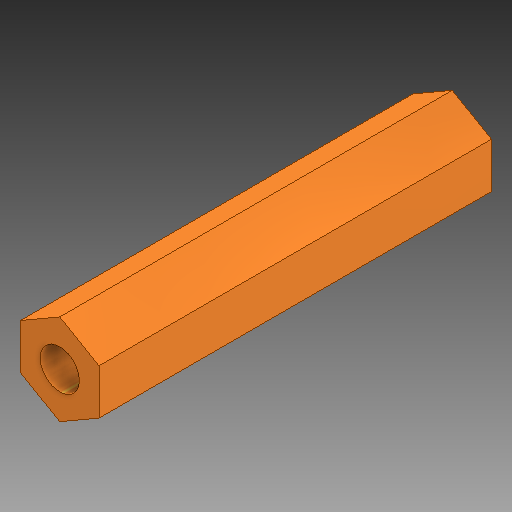
# Autodesk Inventor part: Стойка м3х40
Saved by Autodesk Inventor 2022 (Build 260153000, 153)
## iProperties
Created: 2025-01-23
Part Number: Стойка м3х40
Material: Типовые
Document SubType Name: Modeling
Designer: Ivan
Density: 1 g/cm^3
Appearance: Металл — 1600F
Mass: 0.72325 g
Surface Area: 9.54498 cm^2
Volume: 0.72325 cm^3
Author: Ivan
Title: Стойка м3х40
Autodesk Inventor part; units mm, degrees
ref_plane "YZ Plane" through (0, 0, 0) normal (1, 0, 0) x (0, 1, 0)
ref_plane "XZ Plane" through (0, 0, 0) normal (0, 1, 0) x (-1, 0, 0)
ref_plane "XY Plane" through (0, 0, 0) normal (0, 0, 1) x (1, 0, 0)
sketch "Эскиз1" plane through (0, 0, 0) normal (0, 0, 1) x (1, 0, 0)
  line L0 (0, 3.4641) -> (3, 1.7321)
  line L1 (3, 1.7321) -> (3, -1.7321)
  line L2 (3, -1.7321) -> (0, -3.4641)
  line L3 (0, -3.4641) -> (-3, -1.7321)
  line L4 (-3, -1.7321) -> (-3, 1.7321)
  line L5 (-3, 1.7321) -> (0, 3.4641)
  circle A0 centre (0, 0) radius 1.5
  dimension "d0" = 3
  dimension "d1" = 6
  constraints: 12 end point, 2 coincident, 1 centre point, 1 vertical, 13 other
  measures "d0" diameter of A0
  measures "d1" distance between parallel lines of L4 L1
extrude "Выдавливание1" add sketch "Эскиз1" along normal mid plane 30
